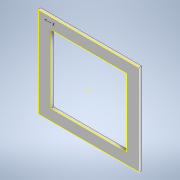
# Autodesk Inventor part: EngravingJigBottom
Saved by Autodesk Inventor 2021 (Build 250183000, 183)
## iProperties
Created: 2021-02-01
Part Number: EngravingJigBottom
Material: Generic
Document SubType Name: Modeling
Designer: Viktor
Density: 1 g/cm^3
Appearance: Default
Author: Viktor
Autodesk Inventor part; units mm, degrees
ref_plane "YZ Plane" through (0, 0, 0) normal (1, 0, 0) x (0, 1, 0)
ref_plane "XZ Plane" through (0, 0, 0) normal (0, 1, 0) x (-1, 0, 0)
ref_plane "XY Plane" through (0, 0, 0) normal (0, 0, 1) x (1, 0, 0)
sketch "Sketch1" plane through (0, 0, 0) normal (0, 0, 1) x (1, 0, 0)
  line L0 (-83.5, -75) -> (83.5, -75)
  line L1 (83.5, -75) -> (83.5, 75)
  line L2 (83.5, 75) -> (-83.5, 75)
  line L3 (-83.5, 75) -> (-83.5, -75)
  line L4 (-83.5, -75) -> (83.5, 75) construction
  line L5 (83.5, -75) -> (-83.5, 75) construction
  line L6 (-111.3333, -100) -> (111.3333, -100)
  line L7 (111.3333, -100) -> (111.3333, 100)
  line L8 (111.3333, 100) -> (-111.3333, 100)
  line L9 (-111.3333, 100) -> (-111.3333, -100)
  line L10 (-111.3333, -100) -> (111.3333, 100) construction
  line L11 (111.3333, -100) -> (-111.3333, 100) construction
  point P0 (0, 0)
  dimension "d0" = 167
  dimension "d1" = 150
  dimension "d2" = 200
  constraints: 24 end point, 4 midpoint, 4 parallel, 2 horizontal, 2 perpendicular, 1 point on line
  measures "d0" distance of L1.end L2.end
  measures "d1" distance of L2.end L0.start
  measures "d2" distance between parallel lines of L6 L8
extrude "Extrusion1" add sketch "Sketch1" along normal blind 6
sketch "Sketch2" plane through (0, 0, 6) normal (0, 0, 1) x (1, 0, 0)
  line L0 (-97.7815, 91.4101) -> (-75.2386, 91.4101) construction
  line L1 (-75.2386, 91.4101) -> (-75.2386, 85.3601) construction
  line L2 (-75.2386, 85.3601) -> (-97.7815, 85.3601) construction
  line L3 (-97.7815, 85.3601) -> (-97.7815, 91.4101) construction
  line L4 (111.3333, -100) -> (111.3333, 100) projected
  line L5 (111.3333, 100) -> (-111.3333, 100) projected
  line L6 (-111.3333, 100) -> (-111.3333, -100) projected
  line L7 (-111.3333, -100) -> (111.3333, -100) projected
  line L8 (-83.5, -75) -> (-83.5, 75) projected
  line L9 (-83.5, 75) -> (83.5, 75) projected
  line L10 (83.5, 75) -> (83.5, -75) projected
  line L11 (83.5, -75) -> (-83.5, -75) projected
  point P0 (0, 0)
  constraints: 2 other
body "Solid1"
